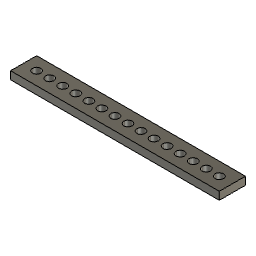
Quadrupedalism_Leg (Autodesk Fusion 360 design; units mm, degrees)
Autodesk Fusion 360 part; units mm, degrees
sketch "Sketch2" plane through (0, 0, 0) normal (0, 0, 1) x (1, 0, 0)
  circle A0 centre (0, 0) radius 1.6
  line L0 (-5, 5) -> (75, 5)
  line L1 (75, 5) -> (75, -5)
  line L2 (75, -5) -> (-5, -5)
  line L3 (-5, -5) -> (-5, 5)
  line L4 (-5, 0) -> (75, 0) construction
  circle A1 centre (5, 0) radius 1.6
  circle A2 centre (10, 0) radius 1.6
  circle A3 centre (15, 0) radius 1.6
  circle A4 centre (20, 0) radius 1.6
  circle A5 centre (25, 0) radius 1.6
  circle A6 centre (30, 0) radius 1.6
  circle A7 centre (35, 0) radius 1.6
  circle A8 centre (40, 0) radius 1.6
  circle A9 centre (45, 0) radius 1.6
  circle A10 centre (50, 0) radius 1.6
  circle A11 centre (55, 0) radius 1.6
  circle A12 centre (60, 0) radius 1.6
  circle A13 centre (65, 0) radius 1.6
  circle A14 centre (70, 0) radius 1.6
  dimension "d46" = 3.2
  dimension "d47" = 80
  dimension "d48" = 10
  dimension "d49" = 5
  dimension "d52" = 5
  dimension "d53" = 0
  constraint coincident A0.centre origin
  constraint horizontal L0
  constraint vertical L1
  constraint horizontal L2
  constraint vertical L3
  constraint midpoint L3 L4.start
  constraint midpoint L1 L4.end
  constraint coincident A0.centre L4
  measures "d46" diameter of A0
  measures "d47" distance of L0.start L0.end
  measures "d48" distance of L0.start L2.end
  measures "d49" distance of A0.centre L3
extrude "Extrude2" add sketch "Sketch2" along normal blind 3
equation "d46 = HoleDiameter"
equation "d47 = LegLength"
equation "d48 = LegWidth"
equation "d49 = HoleSpacing"
equation "d50 = LegLength / HoleSpacing - 1"
equation "d52 = HoleSpacing"
equation "d54 = Thickness"
equation "HoleDiameter = 3.2 mm"
equation "Thickness = 3 mm"
equation "HoleSpacing = 5 mm"
equation "LegWidth = 10 mm"
equation "LegLength = 80 mm"
